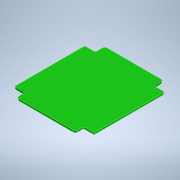
# Autodesk Inventor part: MainBoard
Saved by Autodesk Inventor 2021 (Build 250183000, 183)
## iProperties
Created: 2021-05-13
Part Number: MainBoard
Material: Generic
Document SubType Name: Modeling
Designer: ermoz
Density: 1 g/cm^3
Appearance: Default
Author: ermoz
Autodesk Inventor part; units mm, degrees
ref_plane "YZ Plane" through (0, 0, 0) normal (1, 0, 0) x (0, 1, 0)
ref_plane "XZ Plane" through (0, 0, 0) normal (0, 1, 0) x (-1, 0, 0)
ref_plane "XY Plane" through (0, 0, 0) normal (0, 0, 1) x (1, 0, 0)
sketch "Sketch1" plane through (0, 0, 0) normal (0, 1, 0) x (-1, 0, 0)
  line L0 (-25, -37.5) -> (25, -37.5)
  line L1 (25, -37.5) -> (25, 37.5)
  line L2 (25, 37.5) -> (-25, 37.5)
  line L3 (-25, 37.5) -> (-25, -37.5)
  line L4 (-25, -37.5) -> (25, 37.5) construction
  line L5 (25, -37.5) -> (-25, 37.5) construction
  point P0 (0, 0)
  dimension "d0" = 75
  dimension "d1" = 50
  constraints: 12 end point, 2 midpoint, 2 parallel, 1 horizontal, 1 perpendicular
  measures "d0" distance of L0.end L1.end
  measures "d1" distance of L1.end L2.end
extrude "Extrusion1" add sketch "Sketch1" along normal blind 1.6
fillet "Fillet1" radius 2 4 edges at (-25, 0.8, -37.5) (25, 0.8, -37.5) (25, 0.8, 37.5) (-25, 0.8, 37.5)
sketch "Sketch2" plane through (0, 0, 0) normal (0, -1, 0) x (1, 0, 0)
  line L0 (25, 35.5) -> (25, -35.5) projected
  line L1 (25, -29.5) -> (34, -29.5)
  line L2 (34, -29.5) -> (34, 30.5)
  line L3 (34, 30.5) -> (25, 30.5)
  line L4 (25, 30.5) -> (25, -29.5)
  line L5 (-25, -35.5) -> (-25, 35.5) projected
  line L6 (-25, -29.5) -> (-34, -29.5)
  line L7 (-34, -29.5) -> (-34, 30.5)
  line L8 (-34, 30.5) -> (-25, 30.5)
  line L9 (-25, 30.5) -> (-25, -29.5)
  line L10 (-23, 37.5) -> (23, 37.5) projected
  line L11 (23, -37.5) -> (-23, -37.5) projected
  point P0 (0, 0)
  point P1 (25, 30.5)
  point P2 (-25, 30.5)
  dimension "d5" = 9
  dimension "d6" = 9
  dimension "d7" = 7
  dimension "d8" = 8
  constraints: 16 end point, 4 parallel, 4 point on line, 2 horizontal, 2 perpendicular
  measures "d5" distance of L3.end L2.end
  measures "d6" distance of L7.end L8.end
  measures "d7" distance between parallel lines of L8 L10
  measures "d8" distance between parallel lines of L11 L6
extrude "Extrusion2" add sketch "Sketch2" against normal up to surface (1.6 mm away)
fillet "Fillet2" radius 1 8 edges at (-34, 0.8, 30.5) (-25, 0.8, 30.5) (-25, 0.8, -29.5) (-34, 0.8, -29.5) (25, 0.8, -29.5) (34, 0.8, -29.5) (25, 0.8, 30.5) (34, 0.8, 30.5)
body "Solid1"
